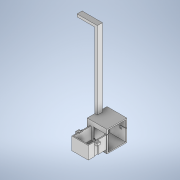
# Autodesk Inventor part: shell 5.0
Saved by Autodesk Inventor 2020.2 (Build 242310000, 310)
## iProperties
Created: 2020-02-13
Part Number: shell 5.0
Material: Generic
Document SubType Name: Modeling
Designer: ColinP
Density: 1 g/cm^3
Appearance: Default
Author: ColinP
Autodesk Inventor part; units mm, degrees
ref_plane "YZ Plane" through (0, 0, 0) normal (1, 0, 0) x (0, 1, 0)
ref_plane "XZ Plane" through (0, 0, 0) normal (0, 1, 0) x (-1, 0, 0)
ref_plane "XY Plane" through (0, 0, 0) normal (0, 0, 1) x (1, 0, 0)
sketch "Sketch1" plane through (0, 0, 0) normal (0, 1, 0) x (-1, 0, 0)
  line L0 (9.2107, 7.1553) -> (-19.7893, 7.1553)
  line L1 (-19.7893, 7.1553) -> (-19.7893, -27.8447)
  line L2 (-19.7893, -27.8447) -> (9.2107, -27.8447)
  line L3 (9.2107, -27.8447) -> (9.2107, 7.1553)
  line L4 (9.2107, 7.1553) -> (11.2107, 7.1553)
  line L5 (11.2107, 7.1553) -> (11.2107, 9.1553)
  line L6 (11.2107, 9.1553) -> (-21.7893, 9.1553)
  line L7 (-21.7893, 9.1553) -> (-21.7893, -29.8447)
  line L8 (-21.7893, -29.8447) -> (11.2107, -29.8447)
  line L9 (11.2107, -29.8447) -> (11.2107, 7.1553)
  point P0 (0, 0)
  dimension "d0" = 29
  dimension "d1" = 35
  dimension "d2" = 2
  dimension "d3" = 2
  dimension "d4" = 33
  dimension "d5" = 39
  constraints: 20 end point, 5 perpendicular, 3 parallel, 2 horizontal, 1 point on line
  measures "d0" distance of L2.end L1.end
  measures "d1" distance of L1.end L0.end
  measures "d2" distance of L0.start L4.end
  measures "d3" distance of L4.end L5.end
  measures "d4" distance of L5.end L6.end
  measures "d5" distance of L6.end L7.end
extrude "Extrusion1" add sketch "Sketch1" along normal blind 2 contours L3 L2 L1 L0
extrude "Extrusion2" add sketch "Sketch1" along normal blind 40
sketch "Sketch2" plane through (21.7893, 0, -29.8447) normal (1, 0, 0) x (0, 0, -1)
  line L0 (-37, 2) -> (-37, 40) projected
  line L1 (-37, 40) -> (-37, 2)
  line L2 (-2, 2) -> (-2, 40) projected
  line L3 (-37, 2) -> (-2, 2)
  line L4 (-2, 2) -> (-2, 40)
  line L5 (-37, 40) -> (-2, 40) projected
  line L6 (-2, 40) -> (-37, 40)
  constraints: 8 end point, 2 collinear, 2 perpendicular
extrude "Extrusion3" cut sketch "Sketch2" against normal blind 10
sketch "Sketch3" plane through (-9.2107, 2, -27.8447) normal (1, 0, 0) x (0, 0, -1)
  line L0 (0, 0) -> (0, 38) projected
  line L1 (0, 0) -> (0, 4.2)
  line L2 (0, 4.2) -> (-4.475, 4.2)
  line L3 (-35, 0) -> (-35, 38) projected
  line L4 (-4.475, 4.2) -> (-30.525, 4.2)
  line L5 (-30.525, 4.2) -> (-30.525, 33.8)
  line L6 (-30.525, 33.8) -> (-4.475, 33.8)
  line L7 (-4.475, 33.8) -> (-4.475, 4.2)
  point P0 (-27.8447, -2)
  dimension "d12" = 4.2
  dimension "d13" = 4.475
  dimension "d14" = 26.05
  dimension "d15" = 29.6
  constraints: 12 end point, 2 parallel, 2 perpendicular, 1 horizontal, 1 point on line
  measures "d12" distance of L0.start L1.end
  measures "d13" distance of L1.end L2.end
  measures "d14" distance of L5.end L6.end
  measures "d15" distance of L4.end L5.end
hole "Hole1" at (-9.2107, 35.8, 2.6803) at (-9.2107, 35.8, -23.3697) at (-9.2107, 6.2, -23.3697) at (-9.2107, 6.2, 2.6803) direction (-1, 0, 0) diameter 3.4 end through all clearance for "Flat Head Machine Screw" size "M3" standard "Ansi Metric M Profile"
sketch "Sketch4" plane through (-11.2107, 2, -27.8447) normal (1, 0, 0) x (0, 0, -1)
  line L0 (-37, 38) -> (-35, 38) projected
  line L1 (-37, 38) -> (2, 38)
  line L2 (2, 38) -> (2, 40)
  line L3 (2, 40) -> (-37, 40)
  line L4 (-37, 40) -> (-37, 38)
  point P0 (-27.8447, -2)
  dimension "d23" = 39
  dimension "d24" = 2
  constraints: 8 end point, 2 parallel, 1 horizontal, 1 perpendicular
  measures "d23" distance of L3.end L2.end
  measures "d24" distance of L2.end L1.end
extrude "Extrusion4" add sketch "Sketch4" along normal blind 33
sketch "Sketch5" plane through (21.7893, 0, 9.1553) normal (1, 0, 0) x (0, 0, -1)
  point P0 (9.1553, 0)
sketch "Sketch6" plane through (-11.2107, 0, -29.8447) normal (-1, 0, 0) x (0, 0, 1)
  point P0 (29.8447, 0)
sketch "Sketch7" plane through (-11.2107, 0, -29.8447) normal (-1, 0, 0) x (0, 0, 1)
  circle A0 centre (6.475, 6.2) radius 1.7 projected
  circle A1 centre (32.525, 35.8) radius 1.7 projected
  circle A2 centre (6.475, 35.8) radius 1.7 projected
  circle A3 centre (32.525, 6.2) radius 1.7 projected
  line L0 (0, 0) -> (39, 0) projected
  line L1 (39, 0) -> (39, 42) projected
  line L2 (0, 42) -> (39, 42) projected
  line L3 (0, 0) -> (0, 42) projected
  circle A4 centre (6.475, 6.2) radius 1.7 projected
  circle A5 centre (6.475, 6.2) radius 3.5
  circle A6 centre (6.475, 35.8) radius 3.5
  circle A7 centre (32.525, 35.8) radius 3.5
  circle A8 centre (32.525, 6.2) radius 1.7 projected
  circle A9 centre (32.525, 6.2) radius 3.5
  point P0 (29.8447, 0)
  dimension "d27" = 7
  dimension "d28" = 7
  dimension "d29" = 7
  dimension "d30" = 7
  constraints: 4 centre point, 4 coincident
  measures "d27" diameter of A5
  measures "d28" diameter of A6
  measures "d29" diameter of A7
  measures "d30" diameter of A9
extrude "Extrusion5" add sketch "Sketch7" along normal blind 5 contours L3 L2 L1 L0
sketch "Sketch8" plane through (21.7893, 0, 9.1553) normal (0, 0, 1) x (1, 0, 0)
  line L0 (0, 0) -> (0, 42) projected
  line L1 (0, 42) -> (0, 32)
  line L2 (0, 32) -> (-3.5, 32)
  line L3 (-3.5, 32) -> (-3.5, 12)
  line L4 (-3.5, 32) -> (16.5, 32) construction
  line L5 (-3.5, 12) -> (-26, 12)
  line L6 (-26, 12) -> (-26, 32)
  line L7 (-26, 32) -> (-3.5, 32)
  point P0 (-21.7893, 0)
  dimension "d33" = 10
  dimension "d34" = 3.5
  dimension "d35" = 20
  dimension "d36" = 90
  dimension "d37" = 22.5
  constraints: 14 end point, 5 perpendicular, 1 horizontal, 1 point on line, 1 vertical
  measures "d33" distance of L0.end L1.end
  measures "d34" distance of L1.end L2.end
  measures "d35" distance of L2.end L3.end
  measures "d36" angle of L3 L4
  measures "d37" distance of L3.end L5.end
extrude "Extrusion6" cut sketch "Sketch8" against normal blind 10
sketch "Sketch9" plane through (21.7893, 0, 9.1553) normal (0, 0, 1) x (1, 0, 0)
  line L0 (-26, 32) -> (-3.5, 32) projected
  line L1 (-26, 32) -> (-26, 33)
  line L2 (-26, 33) -> (0, 33)
  line L3 (0, 2) -> (0, 40) projected
  line L4 (0, 32) -> (-10.0622, 32)
  point P0 (-21.7893, 0)
  dimension "d40" = 1
  constraints: 6 end point, 2 point on line, 1 horizontal, 1 perpendicular, 1 vertical
  measures "d40" distance of L0.start L1.end
extrude "Extrusion7" cut sketch "Sketch9" against normal blind 10
sketch "Sketch10" plane through (-16.2107, 42, 9.1553) normal (0, 0, 1) x (1, 0, 0)
  line L0 (38, -10) -> (34.5, -10) projected
  line L1 (38, -10) -> (38, -34)
  line L2 (38, -40) -> (38, -10) projected
  line L3 (0, -42) -> (0, 0) projected
  line L4 (38, -34) -> (7.52, -34)
  line L5 (7, -40) -> (7, -2) projected
  line L6 (7.52, -34) -> (7.52, -10)
  line L7 (7.52, -10) -> (38, -10)
  line L8 (38, -34) -> (38, -35)
  line L9 (38, -35) -> (6.52, -35)
  line L10 (6.52, -35) -> (6.52, -9)
  line L11 (6.52, -9) -> (38, -9)
  line L12 (38, -2) -> (38, -40) projected
  line L13 (38, -10) -> (38, -9)
  point P0 (16.2107, -42)
  dimension "d43" = 24
  dimension "d44" = 30.48
  dimension "d45" = 1
  dimension "d46" = 31.48
  dimension "d47" = 26
  constraints: 18 end point, 4 perpendicular, 3 point on line, 2 collinear, 1 horizontal
  measures "d43" distance of L0.start L1.end
  measures "d44" distance of L1.end L4.end
  measures "d45" distance of L1.end L8.end
  measures "d46" distance of L8.end L9.end
  measures "d47" distance of L9.end L10.end
extrude "Extrusion8" add sketch "Sketch10" along normal blind 34 contours L0 L7 L6 L4 L2 L9 L5 L11 L12 | L5 L9 L10 L11
sketch "Sketch11" plane through (-9.6907, 9, 9.1553) normal (1, 0, 0) x (0, 0, -1)
  line L0 (-34, -2) -> (-34, -1) projected
  line L1 (-34, -2) -> (-35, -2)
  line L2 (-35, -2) -> (-35, 24)
  line L3 (0, 24) -> (-34, 24) projected
  line L4 (-35, 24) -> (-34, 24)
  line L5 (-34, 24) -> (-34, -2)
  point P0 (9.1553, -9)
  point P1 (0, 26)
  point P2 (-34, -1)
  dimension "d50" = 1
  constraints: 8 end point, 2 perpendicular, 1 horizontal, 1 vertical, 1 other
  measures "d50" distance of L0.start L1.end
extrude "Extrusion9" add sketch "Sketch11" along normal blind 29.48
sketch "Sketch16" plane through (-9.6907, 7, 9.1553) normal (0, -1, 0) x (1, 0, 0)
  line L0 (0, 35) -> (29.48, 35) projected
  line L1 (29.48, 35) -> (30.48, 35)
  line L2 (30.48, 35) -> (30.48, 0)
  line L3 (30.48, 0) -> (29.48, 0)
  line L4 (29.48, 0) -> (29.48, 35)
  point P0 (9.6907, -9.1553)
  dimension "d69" = 1
  dimension "d70" = 35
  constraints: 8 end point, 2 parallel, 1 horizontal, 1 perpendicular
  measures "d69" distance of L2.end L3.end
  measures "d70" distance of L1.end L2.end
extrude "Extrusion14" add sketch "Sketch16" against normal blind 26
sketch "Sketch17" plane through (-4.2107, 33, 9.1553) normal (0, 1, 0) x (1, 0, 0)
  line L0 (24, 0) -> (24, -34) projected
  line L1 (-4.48, -34) -> (24, -34) projected
  line L2 (24, -34) -> (-4.48, -34)
  line L3 (-4.48, 0) -> (-4.48, -34) projected
  line L4 (-4.48, -34) -> (-4.48, 0)
  line L5 (-4.48, 0) -> (26, 0)
  line L6 (25, -34) -> (25, 0) projected
  line L7 (0, 0) -> (26, 0) projected
  line L8 (-5.48, 0) -> (0, 0) projected
  line L9 (-5.48, 0) -> (-5.48, -35) projected
  line L10 (-5.48, -35) -> (25, -35) projected
  line L11 (25, -35) -> (25, -34) projected
  line L12 (26, -34) -> (25, -34) projected
  line L13 (26, 0) -> (26, -34) projected
  point P0 (4.2107, 9.1553)
  constraints: 6 end point, 1 collinear, 1 perpendicular, 1 other
extrude "Extrusion15" cut sketch "Sketch17" against normal blind 10 contours L0 L1 L3 L5
sketch "Sketch18" plane through (-9.6907, 33, 44.1553) normal (0, 1, 0) x (1, 0, 0)
  line L0 (1, 1) -> (1, 35) projected
  line L1 (0, 35) -> (1, 35) projected
  line L2 (0, 35) -> (0, 0) projected
  line L3 (0, 0) -> (30.48, 0) projected
  line L4 (30.48, 0) -> (30.48, 1) projected
  line L5 (29.48, 1) -> (1, 1) projected
  line L6 (31.48, 1) -> (30.48, 1) projected
  line L7 (31.48, 35) -> (31.48, 1) projected
  line L8 (29.48, 35) -> (29.48, 1) projected
  line L9 (29.48, 35) -> (31.48, 35) projected
  point P0 (9.6907, 44.1553)
extrude "Extrusion16" cut sketch "Sketch18" against normal blind 1
sketch "Sketch19" plane through (21.7893, 0, 9.1553) normal (1, 0, 0) x (0, 0, -1)
  line L0 (0, 0) -> (0, 7) projected
  line L1 (0, 0) -> (39, 0) projected
  line L2 (39, 0) -> (39, 42) projected
  line L3 (39, 42) -> (0, 42) projected
  line L4 (0, 33) -> (0, 42) projected
  line L5 (0, 33) -> (2, 33) projected
  line L6 (2, 33) -> (2, 40) projected
  line L7 (2, 40) -> (37, 40) projected
  line L8 (37, 40) -> (37, 2) projected
  line L9 (37, 2) -> (2, 2) projected
  line L10 (2, 2) -> (2, 32) projected
  line L11 (2, 32) -> (0, 32) projected
  line L12 (0, 8) -> (0, 32) projected
  line L13 (0, 8) -> (-34, 8) projected
  line L14 (-34, 7) -> (-34, 8) projected
  line L15 (0, 7) -> (-34, 7) projected
  line L16 (0, 7) -> (0, 8)
  line L17 (0, 0) -> (0, 42) projected
  point P0 (9.1553, 0)
  constraints: 2 end point, 1 collinear
extrude "Extrusion17" add sketch "Sketch19" along normal blind 1 contours L0 L16 L12 L11 L10 L9 L8 L7 L6 L5 L4 L3 L2 L1
sketch "Sketch20" plane through (-9.6907, 32, 44.1553) normal (0, 1, 0) x (1, 0, 0)
  line L0 (29.48, 1) -> (1, 1) projected
  line L1 (15.24, 1) -> (15.24, 15)
  line L2 (15.24, 15) -> (32.74, 15)
  line L3 (32.74, 15) -> (-2.26, 15)
  line L4 (1, 35) -> (1, 1) projected
  line L5 (1, 15) -> (1, 11.5)
  line L6 (1, 11.5) -> (-6, 11.5)
  line L7 (-6, 11.5) -> (-6, 18.5)
  line L8 (-6, 18.5) -> (1, 18.5)
  line L9 (1, 11.5) -> (1, 18.5)
  line L10 (29.48, 1) -> (29.48, 35) projected
  line L11 (29.48, 18.5) -> (36.48, 18.5)
  line L12 (36.48, 18.5) -> (36.48, 11.5)
  line L13 (36.48, 11.5) -> (29.48, 11.5)
  circle A0 centre (-2.26, 15) radius 1.7
  circle A1 centre (32.74, 15) radius 1.7
  point P0 (9.6907, 44.1553)
  point P1 (30.48, 1)
  dimension "d79" = 14
  dimension "d80" = 17.5
  dimension "d81" = 90
  dimension "d82" = 35
  dimension "d83" = 3.5
  dimension "d84" = 7
  dimension "d85" = 7
  dimension "d86" = 7
  dimension "d87" = 3.4
  dimension "d88" = 3.4
  constraints: 22 end point, 11 point on line, 5 perpendicular, 2 centre point, 2 coincident, 1 midpoint, 1 vertical
  measures "d79" distance of L1.start L1.end
  measures "d80" distance of L1.end L2.end
  measures "d81" angle of L1 L2
  measures "d82" distance of L2.end L3.end
  measures "d83" distance of L5.start L5.end
  measures "d84" distance of L5.end L6.end
  measures "d85" distance of L6.end L7.end
  measures "d86" distance of L11.start L11.end
  measures "d87" diameter of A0
  measures "d88" diameter of A1
extrude "Extrusion18" add sketch "Sketch20" against normal blind 5 contours L10 L11 L12 L13 | L6 L7 L8 L4
sketch "Sketch21" plane through (-8.6907, 32, 43.1553) normal (0, 1, 0) x (1, 0, 0)
  line L0 (29.48, 17.5) -> (29.48, 10.5) projected
  line L1 (29.48, 17.5) -> (28.48, 17.5)
  line L2 (28.48, 0) -> (28.48, 34) projected
  line L3 (35.48, 10.5) -> (29.48, 10.5) projected
  line L4 (29.48, 10.5) -> (28.48, 10.5)
  line L5 (28.48, 10.5) -> (28.48, 17.5)
  line L6 (-1, 17.5) -> (-7, 17.5) projected
  line L7 (-1, 17.5) -> (0, 17.5)
  line L8 (0, 34) -> (0, 0) projected
  line L9 (-1, 10.5) -> (-1, 17.5)
  line L10 (-1, 34) -> (-1, -1) projected
  line L11 (-1, -1) -> (-1, 10.5) projected
  line L12 (-1, 10.5) -> (0, 10.5)
  line L13 (0, 10.5) -> (0, 17.5)
  line L14 (29.48, 10.5) -> (29.48, -1) projected
  line L15 (26.98, 36) -> (31.48, 36) projected
  line L16 (26.98, 34) -> (26.98, 36) projected
  line L17 (28.48, 34) -> (26.98, 34) projected
  line L18 (0, 34) -> (0, 0) projected
  line L19 (-1, 34) -> (0, 34) projected
  line L20 (-1, 17.5) -> (-1, 34) projected
  line L21 (-1, 17.5) -> (-7, 17.5) projected
  line L22 (-7, 17.5) -> (-7, 10.5) projected
  line L23 (-7, 10.5) -> (-1, 10.5) projected
  line L24 (-1, -1) -> (-1, 10.5) projected
  line L25 (29.48, -1) -> (-1, -1) projected
  line L26 (31.48, 34) -> (29.48, 34) projected
  line L27 (31.48, 36) -> (31.48, 34) projected
  line L28 (28.48, 0) -> (28.48, 34) projected
  line L29 (0, 0) -> (28.48, 0) projected
  line L30 (29.48, 10.5) -> (35.48, 10.5) projected
  line L31 (35.48, 10.5) -> (35.48, 17.5) projected
  line L32 (35.48, 17.5) -> (29.48, 17.5) projected
  line L33 (29.48, 34) -> (29.48, 17.5) projected
  point P0 (8.6907, 43.1553)
  point P1 (30.1371, 10.5)
  point P2 (29.48, 17.5)
  point P3 (-7, 17.5)
  constraints: 14 end point, 5 point on line, 2 horizontal, 2 perpendicular, 1 collinear
extrude "Extrusion19" cut sketch "Sketch21" against normal blind 1 contours L32 L31 L3 L0 | L0 L4 L2 L1 | L23 L22 L6 L9 | L9 L7 L8 L12
sketch "Sketch30" plane through (20.7893, 7, 44.1553) normal (1, 0, 0) x (0, 0, -1)
  line L0 (11.5, 25) -> (0, 25) projected
  line L1 (0, 0) -> (0, 25) projected
  line L2 (1, 0) -> (0, 0) projected
  line L3 (1, 0) -> (0, 0) projected
  line L4 (35, 0) -> (37, 0)
  line L5 (1, 1) -> (1, 0) projected
  line L6 (35, 1) -> (1, 1) projected
  line L7 (35, 25) -> (35, 1) projected
  line L8 (35, 25) -> (18.5, 25) projected
  line L9 (18.5, 24) -> (18.5, 20) projected
  line L10 (18.5, 20) -> (11.5, 20) projected
  line L11 (11.5, 20) -> (11.5, 24) projected
  line L12 (18.5, 25) -> (18.5, 24) projected
  line L13 (11.5, 24) -> (11.5, 25) projected
  line L14 (18.5, 20) -> (18.5, 0)
  line L15 (35, 0) -> (0, 0) projected
  line L16 (11.5, 20) -> (18.5, 20) projected
  line L17 (11.5, 20) -> (11.5, 0)
  line L18 (35, 1) -> (1, 1) projected
  line L19 (11.5, 1) -> (11.5, 0)
  line L20 (35, 0) -> (1, 0) projected
  line L21 (18.5, 1) -> (18.5, 0)
  point P0 (44.1553, -7)
  constraints: 10 end point, 5 point on line, 2 vertical, 1 parallel, 1 perpendicular
extrude "Extrusion25" add sketch "Sketch30" along normal blind 1 contours L13 L11 L17 L6 L5 L2 L1 L0 | L9 L12 L8 L7 L6 L14
sketch "Sketch31" plane through (-9.6907, 7, 9.1553) normal (-1, 0, 0) x (0, 0, 1)
  line L0 (16.5, 20) -> (16.5, 24) projected
  line L1 (16.5, 25) -> (0, 25) projected
  line L2 (0, 0) -> (0, 25) projected
  line L3 (0, 0) -> (35, 0) projected
  line L4 (35, 25) -> (35, 0) projected
  line L5 (35, 25) -> (23.5, 25) projected
  line L6 (23.5, 24) -> (23.5, 20) projected
  line L7 (23.5, 20) -> (16.5, 20) projected
  line L8 (23.5, 25) -> (23.5, 24) projected
  line L9 (16.5, 24) -> (16.5, 25) projected
  line L10 (0, 0) -> (35, 0) projected
  line L11 (16.5, 20) -> (23.5, 20)
  line L12 (23.5, 20) -> (23.5, 0)
  line L13 (23.5, 0) -> (16.5, 0)
  line L14 (16.5, 0) -> (16.5, 20)
  point P0 (-9.1553, -7)
  point P1 (23.5, 20)
  point P2 (23.5, 0)
  point P3 (16.5, 0)
  constraints: 8 end point, 2 parallel, 1 horizontal, 1 perpendicular, 1 point on line
extrude "Extrusion26" add sketch "Sketch31" along normal blind 1 contours L14 L3 L2 L1 L9 L0 | L6 L8 L5 L4 L3 L12
sketch "Sketch32" plane through (21.7893, 7, 44.1553) normal (0, 0, 1) x (1, 0, 0)
  line L0 (0, 25) -> (-32.48, 25) projected
  line L1 (-32.48, 0) -> (-32.48, 25) projected
  line L2 (-32.48, 0) -> (0, 0) projected
  line L3 (0, 25) -> (0, 0) projected
  point P0 (-21.7893, -7)
extrude "Extrusion27" add sketch "Sketch32" along normal blind 1
sketch "Sketch25" plane through (0, 0, 0) normal (0, -1, 0) x (1, 0, 0)
  line L0 (-16.2107, -29.8447) -> (-16.2107, 9.1553) projected
  line L1 (-16.2107, 9.1553) -> (-16.2107, -5.8447)
  line L2 (-16.2107, -5.8447) -> (-16.2107, -15.8447)
  line L3 (-16.2107, -15.8447) -> (-11.2107, -15.8447)
  line L4 (-11.2107, -15.8447) -> (-11.2107, -5.8447)
  line L5 (-11.2107, -5.8447) -> (-16.2107, -5.8447)
  point P0 (0, 0)
  dimension "d118" = 15
  dimension "d119" = 10
  dimension "d120" = 5
  constraints: 10 end point, 2 perpendicular, 2 point on line, 1 horizontal
  measures "d118" distance of L0.end L1.end
  measures "d119" distance of L1.end L2.end
  measures "d120" distance of L2.end L3.end
extrude "Extrusion21" add sketch "Sketch25" along normal blind 12.7
sketch "Sketch26" plane through (-16.2107, 0, -29.8447) normal (-1, 0, 0) x (0, 0, 1)
  line L0 (24, -12.7) -> (14, -12.7) projected
  line L1 (24, -12.7) -> (24, -7.7)
  line L2 (24, 0) -> (24, -12.7) projected
  line L3 (24, -7.7) -> (14, -7.7)
  line L4 (14, 0) -> (14, -12.7) projected
  line L5 (14, -12.7) -> (14, -7.7)
  point P0 (29.8447, 0)
  dimension "d123" = 5
  constraints: 6 end point, 2 point on line, 1 collinear, 1 perpendicular
  measures "d123" distance of L0.start L1.end
extrude "Extrusion22" add sketch "Sketch26" along normal blind 35
sketch "Sketch27" plane through (-16.2107, 42, 9.1553) normal (0, 1, 0) x (1, 0, 0)
  line L0 (0, 25) -> (0, 15) projected
  line L1 (5, 25) -> (0, 25) projected
  line L2 (0, 25) -> (5, 25)
  line L3 (0, 15) -> (5, 15) projected
  line L4 (5, 25) -> (5, 15)
  line L5 (5, 15) -> (0, 15)
  point P0 (16.2107, 9.1553)
  constraints: 6 end point, 2 perpendicular, 1 horizontal
extrude "Extrusion23" add sketch "Sketch27" along normal blind 152.6502
sketch "Sketch28" plane through (-16.2107, 0, -29.8447) normal (-1, 0, 0) x (0, 0, 1)
  line L0 (14, 194.6502) -> (24, 194.6502) projected
  line L1 (14, 194.6502) -> (14, 189.6502)
  line L2 (14, 42) -> (14, 194.6502) projected
  line L3 (14, 189.6502) -> (24, 189.6502)
  line L4 (24, 42) -> (24, 194.6502) projected
  line L5 (24, 194.6502) -> (14, 194.6502)
  point P0 (29.8447, 0)
  dimension "d128" = 5
  constraints: 6 end point, 2 point on line, 1 parallel, 1 perpendicular
  measures "d128" distance of L0.start L1.end
extrude "Extrusion24" add sketch "Sketch28" along normal blind 35
sketch "Sketch34" plane through (21.7893, 7, 9.1553) normal (1, 0, 0) x (0, 0, -1)
  line L0 (-16.5, 1) -> (-23.5, 1) projected
  line L1 (-23.5, 1) -> (-23.5, 0)
  line L2 (0, 0) -> (-36, 0) projected
  line L3 (-23.5, 1) -> (-23.5, 20) projected
  line L4 (-16.5, 1) -> (-16.5, 20) projected
  line L5 (-23.5, 1) -> (-16.5, 1)
  line L6 (-16.5, 20) -> (-16.5, 0) projected
  line L7 (-16.5, 1) -> (-16.5, 0)
  line L8 (-16.5, 0) -> (-23.5, 0)
  point P0 (9.1553, -7)
  constraints: 8 end point, 2 perpendicular, 1 horizontal, 1 point on line, 1 vertical
extrude "Extrusion28" cut sketch "Sketch34" against normal blind 1
sketch "Sketch35" plane through (-16.2107, 0, -29.8447) normal (0, 0, -1) x (-1, 0, 0)
  line L0 (0, 42) -> (-39, 42) projected
  line L1 (-39, 42) -> (-39, 26)
  line L2 (-39, 0) -> (-39, 42) projected
  line L3 (-39, 26) -> (-29, 26)
  line L4 (-29, 26) -> (-29, 24.5)
  line L5 (-29, 24.5) -> (-27, 24.5)
  line L6 (-27, 24.5) -> (-27, 19.5)
  line L7 (-27, 19.5) -> (-30.5, 19.5)
  line L8 (-30.5, 24.5) -> (-39, 24.5)
  line L9 (-30.5, 19.5) -> (-30.5, 25)
  line L10 (-30.5, 25) -> (-39, 25)
  line L11 (-39, 26) -> (-39, 25)
  point P0 (-16.2107, 0)
  dimension "d139" = 16
  dimension "d140" = 10
  dimension "d141" = 1.5
  dimension "d142" = 2
  dimension "d143" = 5
  dimension "d144" = 3.5
  dimension "d145" = 5.5
  constraints: 20 end point, 6 perpendicular, 5 point on line, 1 horizontal, 1 vertical
  measures "d139" distance of L0.end L1.end
  measures "d140" distance of L1.end L3.end
  measures "d141" distance of L3.end L4.end
  measures "d142" distance of L4.end L5.end
  measures "d143" distance of L5.end L6.end
  measures "d144" distance of L6.end L7.end
  measures "d145" distance of L7.end L9.end
extrude "Extrusion29" cut sketch "Sketch35" against normal blind 10 contours L2 L3 L4 L5 L6 L7 L9 L10
body "Solid1"
